Autodesk Fusion 360 part; units mm, degrees
(part 16 of 21)
extrude "Estrusione10" add sketch "Schizzo9" along normal blind 1 text T0 in component "Spur Gear (60 teeth) (1)"
component "Spur Gear (60 teeth) (1)" placed x (1, 0, 0) y (0, 1, 0) z (0, 0, 1) at (0, 0, 0)

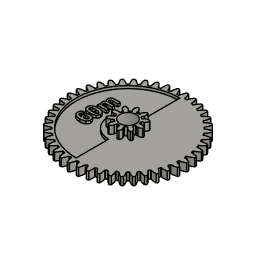
design "6 intermedio ore"
description: Spur Gear; Module: 1.000000; Num Teeth: 44; Pressure Angle: 20.000000; Backlash: 0.00 mm
description: Spur Gear; Module: 1.000000; Num Teeth: 10; Pressure Angle: 20.000000; Backlash: 0.00 mm
Autodesk Fusion 360 part; units mm, degrees
sketch "Schizzo1" plane through (0, 0, 0) normal (0, 0, 1) x (1, 0, 0) in component "Spur Gear (44 teeth)"
  circle A0 centre (0, 0) radius 20.7492
  circle A1 centre (0, 0) radius 3.1
extrude "Estrusione1" add sketch "Schizzo1" along normal blind 3 makes body 1 in component "Spur Gear (44 teeth)"
sketch "Schizzo2" plane through (0, 0, 0) normal (0, 0, 1) x (1, 0, 0) in component "Spur Gear (44 teeth)"
  spline S0 degree 5 poles (20.6468, -1.0457) (20.6535, -1.0457) (20.667, -1.0458) (20.6873, -1.0456) (20.7143, -1.0451) (20.7481, -1.044) (20.7819, -1.0422) (20.8157, -1.04) (20.8495, -1.0372) (20.8833, -1.034) (20.9172, -1.0304) (20.951, -1.0264) (20.9848, -1.022) (21.0187, -1.0174) (21.0525, -1.0125) (21.0863, -1.0073) (21.1202, -1.0019) (21.154, -0.9961) (21.1878, -0.9902) (21.2216, -0.9839) (21.2554, -0.9774) (21.2892, -0.9707) (21.323, -0.9637) (21.3568, -0.9565) (21.3906, -0.9491) (21.4244, -0.9415) (21.4581, -0.9337) (21.4919, -0.9256) (21.5256, -0.9174) (21.5594, -0.9089) (21.5931, -0.9002) (21.6268, -0.8914) (21.6605, -0.8823) (21.6942, -0.8731) (21.7279, -0.8636) (21.7616, -0.854) (21.7952, -0.8442) (21.8289, -0.8343) (21.8625, -0.8241) (21.8961, -0.8138) (21.9298, -0.8033) (21.9634, -0.7926) (21.9969, -0.7817) (22.0305, -0.7707) (22.0641, -0.7595) (22.0976, -0.7481) (22.1311, -0.7366) (22.1646, -0.7249) (22.1981, -0.7131) (22.2316, -0.7011) (22.2651, -0.6889) (22.2985, -0.6766) (22.332, -0.6642) (22.3654, -0.6515) (22.3988, -0.6387) (22.4322, -0.6258) (22.4655, -0.6127) (22.4989, -0.5995) (22.5322, -0.5861) (22.5655, -0.5726) (22.5988, -0.5589) (22.6321, -0.5451) (22.6653, -0.5311) (22.6986, -0.517) (22.7318, -0.5027) (22.765, -0.4883) (22.7982, -0.4738) (22.8313, -0.4591) (22.8645, -0.4443) (22.8976, -0.4294) (22.9307, -0.4143) (22.9571, -0.4021) (22.977, -0.3929) (22.9902, -0.3867) (22.9968, -0.3836) knots 0 0 0 0 0 0 0.01428571 0.02857143 0.04285714 0.05714286 0.07142857 0.08571429 0.1 0.11428571 0.12857143 0.14285714 0.15714286 0.17142857 0.18571429 0.2 0.21428571 0.22857143 0.24285714 0.25714286 0.27142857 0.28571429 0.3 0.31428571 0.32857143 0.34285714 0.35714286 0.37142857 0.38571429 0.4 0.41428571 0.42857143 0.44285714 0.45714286 0.47142857 0.48571429 0.5 0.51428571 0.52857143 0.54285714 0.55714286 0.57142857 0.58571429 0.6 0.61428571 0.62857143 0.64285714 0.65714286 0.67142857 0.68571429 0.7 0.71428571 0.72857143 0.74285714 0.75714286 0.77142857 0.78571429 0.8 0.81428571 0.82857143 0.84285714 0.85714286 0.87142857 0.88571429 0.9 0.91428571 0.92857143 0.94285714 0.95714286 0.97142857 0.98571429 1 1 1 1 1 1
  spline S1 degree 5 poles (20.6468, 1.0457) (20.6535, 1.0457) (20.667, 1.0458) (20.6873, 1.0456) (20.7143, 1.0451) (20.7481, 1.044) (20.7819, 1.0422) (20.8157, 1.04) (20.8495, 1.0372) (20.8833, 1.034) (20.9172, 1.0304) (20.951, 1.0264) (20.9848, 1.022) (21.0187, 1.0174) (21.0525, 1.0125) (21.0863, 1.0073) (21.1202, 1.0019) (21.154, 0.9961) (21.1878, 0.9902) (21.2216, 0.9839) (21.2554, 0.9774) (21.2892, 0.9707) (21.323, 0.9637) (21.3568, 0.9565) (21.3906, 0.9491) (21.4244, 0.9415) (21.4581, 0.9337) (21.4919, 0.9256) (21.5256, 0.9174) (21.5594, 0.9089) (21.5931, 0.9002) (21.6268, 0.8914) (21.6605, 0.8823) (21.6942, 0.8731) (21.7279, 0.8636) (21.7616, 0.854) (21.7952, 0.8442) (21.8289, 0.8343) (21.8625, 0.8241) (21.8961, 0.8138) (21.9298, 0.8033) (21.9634, 0.7926) (21.9969, 0.7817) (22.0305, 0.7707) (22.0641, 0.7595) (22.0976, 0.7481) (22.1311, 0.7366) (22.1646, 0.7249) (22.1981, 0.7131) (22.2316, 0.7011) (22.2651, 0.6889) (22.2985, 0.6766) (22.332, 0.6642) (22.3654, 0.6515) (22.3988, 0.6387) (22.4322, 0.6258) (22.4655, 0.6127) (22.4989, 0.5995) (22.5322, 0.5861) (22.5655, 0.5726) (22.5988, 0.5589) (22.6321, 0.5451) (22.6653, 0.5311) (22.6986, 0.517) (22.7318, 0.5027) (22.765, 0.4883) (22.7982, 0.4738) (22.8313, 0.4591) (22.8645, 0.4443) (22.8976, 0.4294) (22.9307, 0.4143) (22.9571, 0.4021) (22.977, 0.3929) (22.9902, 0.3867) (22.9968, 0.3836) knots 0 0 0 0 0 0 0.01428571 0.02857143 0.04285714 0.05714286 0.07142857 0.08571429 0.1 0.11428571 0.12857143 0.14285714 0.15714286 0.17142857 0.18571429 0.2 0.21428571 0.22857143 0.24285714 0.25714286 0.27142857 0.28571429 0.3 0.31428571 0.32857143 0.34285714 0.35714286 0.37142857 0.38571429 0.4 0.41428571 0.42857143 0.44285714 0.45714286 0.47142857 0.48571429 0.5 0.51428571 0.52857143 0.54285714 0.55714286 0.57142857 0.58571429 0.6 0.61428571 0.62857143 0.64285714 0.65714286 0.67142857 0.68571429 0.7 0.71428571 0.72857143 0.74285714 0.75714286 0.77142857 0.78571429 0.8 0.81428571 0.82857143 0.84285714 0.85714286 0.87142857 0.88571429 0.9 0.91428571 0.92857143 0.94285714 0.95714286 0.97142857 0.98571429 1 1 1 1 1 1
  arc A0 (22.9968, -0.3836) -> (22.9968, 0.3836) centre (0, 0) ccw
  line L0 (20.6468, 1.0457) -> (20.6468, -1.0457)
  point P0 (20.8135, -1.04)
  point P1 (20.9807, -1.0225)
  point P2 (21.1483, -0.9971)
  point P3 (21.3162, -0.9651)
  point P4 (21.4842, -0.9274)
  point P5 (21.6524, -0.8845)
  point P6 (21.8206, -0.8367)
  point P7 (21.9888, -0.7843)
  point P8 (22.1571, -0.7276)
  point P9 (22.3253, -0.6666)
  point P10 (22.4934, -0.6017)
  point P11 (22.6613, -0.5328)
  point P12 (22.8292, -0.4601)
  point P13 (20.8135, 1.04)
  point P14 (20.9807, 1.0225)
  point P15 (21.1483, 0.9971)
  point P16 (21.3162, 0.9651)
  point P17 (21.4842, 0.9274)
  point P18 (21.6524, 0.8845)
  point P19 (21.8206, 0.8367)
  point P20 (21.9888, 0.7843)
  point P21 (22.1571, 0.7276)
  point P22 (22.3253, 0.6666)
  point P23 (22.4934, 0.6017)
  point P24 (22.6613, 0.5328)
  point P25 (22.8292, 0.4601)
extrude "Estrusione2" add sketch "Schizzo2" along normal blind 3 bodies 1 in component "Spur Gear (44 teeth)"
fillet "Raccordo1" radius 0.1 2 edges at (20.7229, 1.0448, 1.5) (20.7229, -1.0448, 1.5) on bodies 1 in component "Spur Gear (44 teeth)"
pattern_circular "Serie C1" count 44 over 360 about axis through (0, 0, 0) along (0, 0, 1) of "Estrusione2", "Raccordo1" in component "Spur Gear (44 teeth)"
sketch "Schizzo3" plane through (0, 0, 0) normal (0, 0, 1) x (1, 0, 0) in component "Spur Gear (44 teeth)"
  circle A0 centre (0, 0) radius 22 construction
sketch "Schizzo1 (2)" plane through (0, 0, 0) normal (0, 0, 1) x (1, 0, 0) in component "Spur Gear (10 teeth)"
  circle A0 centre (0, 0) radius 3.7492
  circle A1 centre (0, 0) radius 3.1
extrude "Estrusione1'" add sketch "Schizzo1 (2)" along normal blind 6 separate body makes body 2 in component "Spur Gear (10 teeth)"
sketch "Schizzo2 (2)" plane through (0, 0, 0) normal (0, 0, 1) x (1, 0, 0) in component "Spur Gear (10 teeth)"
  spline S0 degree 5 poles (4.6291, -0.8041) (4.6329, -0.8047) (4.6405, -0.8059) (4.6519, -0.8073) (4.6672, -0.8084) (4.6864, -0.8088) (4.7057, -0.8085) (4.7251, -0.8077) (4.7445, -0.8066) (4.7639, -0.8054) (4.7834, -0.804) (4.8029, -0.8024) (4.8224, -0.8004) (4.842, -0.7981) (4.8616, -0.7954) (4.8812, -0.7924) (4.9009, -0.7891) (4.9205, -0.7856) (4.9402, -0.7818) (4.9599, -0.7778) (4.9796, -0.7737) (4.9993, -0.7693) (5.019, -0.7646) (5.0388, -0.7598) (5.0585, -0.7547) (5.0783, -0.7493) (5.098, -0.7438) (5.1178, -0.738) (5.1375, -0.7321) (5.1573, -0.7259) (5.177, -0.7196) (5.1968, -0.7131) (5.2165, -0.7063) (5.2363, -0.6994) (5.256, -0.6923) (5.2757, -0.685) (5.2955, -0.6775) (5.3152, -0.6698) (5.3349, -0.6619) (5.3546, -0.6538) (5.3743, -0.6456) (5.394, -0.6372) (5.4136, -0.6286) (5.4333, -0.6198) (5.4529, -0.6109) (5.4725, -0.6018) (5.4921, -0.5925) (5.5117, -0.583) (5.5312, -0.5734) (5.5508, -0.5636) (5.5703, -0.5536) (5.5898, -0.5435) (5.6093, -0.5332) (5.6287, -0.5228) (5.6482, -0.5121) (5.6676, -0.5013) (5.6869, -0.4904) (5.7063, -0.4793) (5.7256, -0.468) (5.7449, -0.4566) (5.7642, -0.445) (5.7834, -0.4332) (5.8026, -0.4213) (5.8218, -0.4093) (5.8409, -0.397) (5.86, -0.3847) (5.8791, -0.3721) (5.8982, -0.3595) (5.9172, -0.3466) (5.9361, -0.3336) (5.9551, -0.3205) (5.9702, -0.3099) (5.9815, -0.3018) (5.989, -0.2964) (5.9928, -0.2937) knots 0 0 0 0 0 0 0.01428571 0.02857143 0.04285714 0.05714286 0.07142857 0.08571429 0.1 0.11428571 0.12857143 0.14285714 0.15714286 0.17142857 0.18571429 0.2 0.21428571 0.22857143 0.24285714 0.25714286 0.27142857 0.28571429 0.3 0.31428571 0.32857143 0.34285714 0.35714286 0.37142857 0.38571429 0.4 0.41428571 0.42857143 0.44285714 0.45714286 0.47142857 0.48571429 0.5 0.51428571 0.52857143 0.54285714 0.55714286 0.57142857 0.58571429 0.6 0.61428571 0.62857143 0.64285714 0.65714286 0.67142857 0.68571429 0.7 0.71428571 0.72857143 0.74285714 0.75714286 0.77142857 0.78571429 0.8 0.81428571 0.82857143 0.84285714 0.85714286 0.87142857 0.88571429 0.9 0.91428571 0.92857143 0.94285714 0.95714286 0.97142857 0.98571429 1 1 1 1 1 1
  spline S1 degree 5 poles (4.6291, 0.8041) (4.6329, 0.8047) (4.6405, 0.8059) (4.6519, 0.8073) (4.6672, 0.8084) (4.6864, 0.8088) (4.7057, 0.8085) (4.7251, 0.8077) (4.7445, 0.8066) (4.7639, 0.8054) (4.7834, 0.804) (4.8029, 0.8024) (4.8224, 0.8004) (4.842, 0.7981) (4.8616, 0.7954) (4.8812, 0.7924) (4.9009, 0.7891) (4.9205, 0.7856) (4.9402, 0.7818) (4.9599, 0.7778) (4.9796, 0.7737) (4.9993, 0.7693) (5.019, 0.7646) (5.0388, 0.7598) (5.0585, 0.7547) (5.0783, 0.7493) (5.098, 0.7438) (5.1178, 0.738) (5.1375, 0.7321) (5.1573, 0.7259) (5.177, 0.7196) (5.1968, 0.7131) (5.2165, 0.7063) (5.2363, 0.6994) (5.256, 0.6923) (5.2757, 0.685) (5.2955, 0.6775) (5.3152, 0.6698) (5.3349, 0.6619) (5.3546, 0.6538) (5.3743, 0.6456) (5.394, 0.6372) (5.4136, 0.6286) (5.4333, 0.6198) (5.4529, 0.6109) (5.4725, 0.6018) (5.4921, 0.5925) (5.5117, 0.583) (5.5312, 0.5734) (5.5508, 0.5636) (5.5703, 0.5536) (5.5898, 0.5435) (5.6093, 0.5332) (5.6287, 0.5228) (5.6482, 0.5121) (5.6676, 0.5013) (5.6869, 0.4904) (5.7063, 0.4793) (5.7256, 0.468) (5.7449, 0.4566) (5.7642, 0.445) (5.7834, 0.4332) (5.8026, 0.4213) (5.8218, 0.4093) (5.8409, 0.397) (5.86, 0.3847) (5.8791, 0.3721) (5.8982, 0.3595) (5.9172, 0.3466) (5.9361, 0.3336) (5.9551, 0.3205) (5.9702, 0.3099) (5.9815, 0.3018) (5.989, 0.2964) (5.9928, 0.2937) knots 0 0 0 0 0 0 0.01428571 0.02857143 0.04285714 0.05714286 0.07142857 0.08571429 0.1 0.11428571 0.12857143 0.14285714 0.15714286 0.17142857 0.18571429 0.2 0.21428571 0.22857143 0.24285714 0.25714286 0.27142857 0.28571429 0.3 0.31428571 0.32857143 0.34285714 0.35714286 0.37142857 0.38571429 0.4 0.41428571 0.42857143 0.44285714 0.45714286 0.47142857 0.48571429 0.5 0.51428571 0.52857143 0.54285714 0.55714286 0.57142857 0.58571429 0.6 0.61428571 0.62857143 0.64285714 0.65714286 0.67142857 0.68571429 0.7 0.71428571 0.72857143 0.74285714 0.75714286 0.77142857 0.78571429 0.8 0.81428571 0.82857143 0.84285714 0.85714286 0.87142857 0.88571429 0.9 0.91428571 0.92857143 0.94285714 0.95714286 0.97142857 0.98571429 1 1 1 1 1 1
  arc A0 (5.9928, -0.2937) -> (5.9928, 0.2937) centre (0, 0) ccw
  line L0 (3.684, -0.6416) -> (4.6291, -0.8041)
  line L1 (3.684, 0.6416) -> (4.6291, 0.8041)
  line L2 (3.684, -0.6416) -> (3.684, 0.6416)
  point P0 (4.7229, -0.8077)
  point P1 (4.8183, -0.8008)
  point P2 (4.9148, -0.7866)
  point P3 (5.0121, -0.7662)
  point P4 (5.11, -0.7403)
  point P5 (5.2082, -0.7091)
  point P6 (5.3067, -0.673)
  point P7 (5.4054, -0.6322)
  point P8 (5.504, -0.5867)
  point P9 (5.6025, -0.5368)
  point P10 (5.7007, -0.4824)
  point P11 (5.7986, -0.4238)
  point P12 (5.896, -0.3609)
  point P13 (4.7229, 0.8077)
  point P14 (4.8183, 0.8008)
  point P15 (4.9148, 0.7866)
  point P16 (5.0121, 0.7662)
  point P17 (5.11, 0.7403)
  point P18 (5.2082, 0.7091)
  point P19 (5.3067, 0.673)
  point P20 (5.4054, 0.6322)
  point P21 (5.504, 0.5867)
  point P22 (5.6025, 0.5368)
  point P23 (5.7007, 0.4824)
  point P24 (5.7986, 0.4238)
  point P25 (5.896, 0.3609)
extrude "Estrusione2'" add sketch "Schizzo2 (2)" along normal blind 6 bodies 2 in component "Spur Gear (10 teeth)"
fillet "Raccordo1'" radius 0.1 2 edges at (3.6936, -0.6433, 3) (3.6936, 0.6433, 3) on bodies 2 in component "Spur Gear (10 teeth)"
pattern_circular "Serie C1'" count 10 over 360 about axis through (0, 0, 0) along (0, 0, 1) of "Estrusione2'", "Raccordo1'" in component "Spur Gear (10 teeth)"
sketch "Schizzo3 (2)" plane through (0, 0, 0) normal (0, 0, 1) x (1, 0, 0) in component "Spur Gear (10 teeth)"
  circle A0 centre (0, 0) radius 5 construction
combine "Combina1" operation add target body 1 tool bodies 2 in component "Spur Gear (44 teeth)"
sketch "Schizzo1 (3)" plane through (0, 0, 3) normal (0, 0, 1) x (-1, 0, 0)
  arc A0 (-3.7907, 0.66) -> (-3.6757, 0.7388) centre (-3.7737, 0.7585) ccw
  arc A1 (-3.408, 1.5628) -> (-3.6757, 0.7388) centre (0, 0) ccw
  arc A2 (-3.408, 1.5628) -> (-3.4546, 1.6942) centre (-3.4988, 1.6045) ccw
  line L0 (-3.4546, 1.6942) -> (-4.2177, 2.0704)
  spline S0 degree 3 poles (-4.2177, 2.0704) (-4.2458, 2.0843) (-4.2713, 2.1025) (-4.3719, 2.1848) (-4.5424, 2.3303) (-4.8488, 2.838) (-4.9461, 3.0593) (-5.0209, 3.2848) knots 0 0 0 0 0.009402 0.009402 0.024238 0.024238 0.034093 0.034093 0.034093 0.034093
  arc A3 (-4.6756, 3.7601) -> (-5.0209, 3.2848) centre (0, 0) ccw
  spline S1 degree 3 poles (-4.6756, 3.7601) (-4.4172, 3.7585) (-4.1552, 3.7302) (-3.7444, 3.6242) (-3.6325, 3.5789) (-3.4729, 3.5079) (-3.34, 3.4408) (-3.2724, 3.3715) knots 0 0 0 0 0.077518 0.077518 0.128006 0.128006 0.19629 0.19629 0.19629 0.19629
  line L1 (-3.2724, 3.3715) -> (-2.6788, 2.762)
  arc A4 (-2.6788, 2.762) -> (-2.5394, 2.7582) centre (-2.6072, 2.8318) ccw
  arc A5 (-1.8385, 3.2675) -> (-2.5394, 2.7582) centre (0, 0) ccw
  arc A6 (-1.8385, 3.2675) -> (-1.799, 3.4012) centre (-1.8875, 3.3546) ccw
  line L2 (-1.799, 3.4012) -> (-2.1952, 4.1541)
  spline S2 degree 3 poles (-2.1952, 4.1541) (-2.2098, 4.1818) (-2.2197, 4.2116) (-2.2528, 4.3373) (-2.3052, 4.5552) (-2.2547, 5.1461) (-2.2033, 5.3822) (-2.1312, 5.6087) knots 0 0 0 0 0.009402 0.009402 0.024238 0.024238 0.034093 0.034093 0.034093 0.034093
  arc A7 (-1.5725, 5.7903) -> (-2.1312, 5.6087) centre (0, 0) ccw
  spline S3 degree 3 poles (-1.5725, 5.7903) (-1.3644, 5.6371) (-1.1691, 5.4601) (-0.899, 5.133) (-0.8351, 5.0306) (-0.7478, 4.8792) (-0.6796, 4.7468) (-0.6658, 4.6511) knots 0 0 0 0 0.077518 0.077518 0.128006 0.128006 0.19629 0.19629 0.19629 0.19629
  line L3 (-0.6658, 4.6511) -> (-0.5437, 3.8091)
  arc A8 (-0.5437, 3.8091) -> (-0.4332, 3.7241) centre (-0.4448, 3.8234) ccw
  arc A9 (0.4332, 3.7241) -> (-0.4332, 3.7241) centre (0, 0) ccw
  arc A10 (0.4332, 3.7241) -> (0.5437, 3.8091) centre (0.4448, 3.8234) ccw
  line L4 (0.5437, 3.8091) -> (0.6658, 4.6511)
  spline S4 degree 3 poles (0.6658, 4.6511) (0.6703, 4.6821) (0.6797, 4.7119) (0.7268, 4.8331) (0.8125, 5.0402) (1.2007, 5.4885) (1.3811, 5.6494) (1.5725, 5.7903) knots 0 0 0 0 0.009402 0.009402 0.024238 0.024238 0.034093 0.034093 0.034093 0.034093
  arc A11 (2.1312, 5.6087) -> (1.5725, 5.7903) centre (0, 0) ccw
  spline S5 degree 3 poles (2.1312, 5.6087) (2.2096, 5.3625) (2.2636, 5.1045) (2.2897, 4.6811) (2.2813, 4.5607) (2.263, 4.3869) (2.2403, 4.2397) (2.1952, 4.1541) knots 0 0 0 0 0.077518 0.077518 0.128006 0.128006 0.19629 0.19629 0.19629 0.19629
  line L5 (2.1952, 4.1541) -> (1.799, 3.4012)
  arc A12 (1.799, 3.4012) -> (1.8385, 3.2675) centre (1.8875, 3.3546) ccw
  arc A13 (2.5394, 2.7582) -> (1.8385, 3.2675) centre (0, 0) ccw
  arc A14 (2.5394, 2.7582) -> (2.6788, 2.762) centre (2.6072, 2.8318) ccw
  line L6 (2.6788, 2.762) -> (3.2724, 3.3715)
  spline S6 degree 3 poles (3.2724, 3.3715) (3.2943, 3.3939) (3.3195, 3.4125) (3.4288, 3.4828) (3.6199, 3.6) (4.1975, 3.7345) (4.438, 3.7587) (4.6756, 3.7601) knots 0 0 0 0 0.009402 0.009402 0.024238 0.024238 0.034093 0.034093 0.034093 0.034093
  arc A15 (5.0209, 3.2848) -> (4.6756, 3.7601) centre (0, 0) ccw
  spline S7 degree 3 poles (5.0209, 3.2848) (4.9396, 3.0396) (4.8316, 2.7991) (4.6039, 2.4412) (4.5263, 2.3488) (4.4094, 2.2189) (4.3045, 2.1132) (4.2177, 2.0704) knots 0 0 0 0 0.077518 0.077518 0.128006 0.128006 0.19629 0.19629 0.19629 0.19629
  line L7 (4.2177, 2.0704) -> (3.4546, 1.6942)
  arc A16 (3.4546, 1.6942) -> (3.408, 1.5628) centre (3.4988, 1.6045) ccw
  arc A17 (3.6757, 0.7388) -> (3.408, 1.5628) centre (0, 0) ccw
  arc A18 (3.6757, 0.7388) -> (3.7907, 0.66) centre (3.7737, 0.7585) ccw
  line L8 (3.7907, 0.66) -> (4.6291, 0.8041)
  spline S8 degree 3 poles (4.6291, 0.8041) (4.66, 0.8094) (4.6914, 0.8096) (4.8211, 0.8023) (5.0446, 0.7847) (5.5909, 0.5541) (5.7997, 0.4323) (5.9928, 0.2937) knots 0 0 0 0 0.009402 0.009402 0.024238 0.024238 0.034093 0.034093 0.034093 0.034093
  arc A19 (5.9928, -0.2937) -> (5.9928, 0.2937) centre (0, 0) ccw
  spline S9 degree 3 poles (5.9928, -0.2937) (5.7828, -0.4443) (5.5541, -0.5754) (5.1596, -0.7311) (5.0424, -0.7603) (4.8715, -0.7966) (4.7245, -0.8205) (4.6291, -0.8041) knots 0 0 0 0 0.077518 0.077518 0.128006 0.128006 0.19629 0.19629 0.19629 0.19629
  line L9 (4.6291, -0.8041) -> (3.7907, -0.66)
  arc A20 (3.7907, -0.66) -> (3.6757, -0.7388) centre (3.7737, -0.7585) ccw
  arc A21 (3.408, -1.5628) -> (3.6757, -0.7388) centre (0, 0) ccw
  arc A22 (3.408, -1.5628) -> (3.4546, -1.6942) centre (3.4988, -1.6045) ccw
  line L10 (3.4546, -1.6942) -> (4.2177, -2.0704)
  spline S10 degree 3 poles (4.2177, -2.0704) (4.2458, -2.0843) (4.2713, -2.1025) (4.3719, -2.1848) (4.5424, -2.3303) (4.8488, -2.838) (4.9461, -3.0593) (5.0209, -3.2848) knots 0 0 0 0 0.009402 0.009402 0.024238 0.024238 0.034093 0.034093 0.034093 0.034093
  arc A23 (4.6756, -3.7601) -> (5.0209, -3.2848) centre (0, 0) ccw
  spline S11 degree 3 poles (4.6756, -3.7601) (4.4172, -3.7585) (4.1552, -3.7302) (3.7444, -3.6242) (3.6325, -3.5789) (3.4729, -3.5079) (3.34, -3.4408) (3.2724, -3.3715) knots 0 0 0 0 0.077518 0.077518 0.128006 0.128006 0.19629 0.19629 0.19629 0.19629
  line L11 (3.2724, -3.3715) -> (2.6788, -2.762)
  arc A24 (2.6788, -2.762) -> (2.5394, -2.7582) centre (2.6072, -2.8318) ccw
  arc A25 (1.8385, -3.2675) -> (2.5394, -2.7582) centre (0, 0) ccw
  arc A26 (1.8385, -3.2675) -> (1.799, -3.4012) centre (1.8875, -3.3546) ccw
  line L12 (1.799, -3.4012) -> (2.1952, -4.1541)
  spline S12 degree 3 poles (2.1952, -4.1541) (2.2098, -4.1818) (2.2197, -4.2116) (2.2528, -4.3373) (2.3052, -4.5552) (2.2547, -5.1461) (2.2033, -5.3822) (2.1312, -5.6087) knots 0 0 0 0 0.009402 0.009402 0.024238 0.024238 0.034093 0.034093 0.034093 0.034093
  arc A27 (1.5725, -5.7903) -> (2.1312, -5.6087) centre (0, 0) ccw
  spline S13 degree 3 poles (1.5725, -5.7903) (1.3644, -5.6371) (1.1691, -5.4601) (0.899, -5.133) (0.8351, -5.0306) (0.7478, -4.8792) (0.6796, -4.7468) (0.6658, -4.6511) knots 0 0 0 0 0.077518 0.077518 0.128006 0.128006 0.19629 0.19629 0.19629 0.19629
  line L13 (0.6658, -4.6511) -> (0.5437, -3.8091)
  arc A28 (0.5437, -3.8091) -> (0.4332, -3.7241) centre (0.4448, -3.8234) ccw
  arc A29 (-0.4332, -3.7241) -> (0.4332, -3.7241) centre (0, 0) ccw
  arc A30 (-0.4332, -3.7241) -> (-0.5437, -3.8091) centre (-0.4448, -3.8234) ccw
  line L14 (-0.5437, -3.8091) -> (-0.6658, -4.6511)
  spline S14 degree 3 poles (-0.6658, -4.6511) (-0.6703, -4.6821) (-0.6797, -4.7119) (-0.7268, -4.8331) (-0.8125, -5.0402) (-1.2007, -5.4885) (-1.3811, -5.6494) (-1.5725, -5.7903) knots 0 0 0 0 0.009402 0.009402 0.024238 0.024238 0.034093 0.034093 0.034093 0.034093
  arc A31 (-2.1312, -5.6087) -> (-1.5725, -5.7903) centre (0, 0) ccw
  spline S15 degree 3 poles (-2.1312, -5.6087) (-2.2096, -5.3625) (-2.2636, -5.1045) (-2.2897, -4.6811) (-2.2813, -4.5607) (-2.263, -4.3869) (-2.2403, -4.2397) (-2.1952, -4.1541) knots 0 0 0 0 0.077518 0.077518 0.128006 0.128006 0.19629 0.19629 0.19629 0.19629
  line L15 (-2.1952, -4.1541) -> (-1.799, -3.4012)
  arc A32 (-1.799, -3.4012) -> (-1.8385, -3.2675) centre (-1.8875, -3.3546) ccw
  arc A33 (-2.5394, -2.7582) -> (-1.8385, -3.2675) centre (0, 0) ccw
  arc A34 (-2.5394, -2.7582) -> (-2.6788, -2.762) centre (-2.6072, -2.8318) ccw
  line L16 (-2.6788, -2.762) -> (-3.2724, -3.3715)
  spline S16 degree 3 poles (-3.2724, -3.3715) (-3.2943, -3.3939) (-3.3195, -3.4125) (-3.4288, -3.4828) (-3.6199, -3.6) (-4.1975, -3.7345) (-4.438, -3.7587) (-4.6756, -3.7601) knots 0 0 0 0 0.009402 0.009402 0.024238 0.024238 0.034093 0.034093 0.034093 0.034093
  arc A35 (-5.0209, -3.2848) -> (-4.6756, -3.7601) centre (0, 0) ccw
  spline S17 degree 3 poles (-5.0209, -3.2848) (-4.9396, -3.0396) (-4.8316, -2.7991) (-4.6039, -2.4412) (-4.5263, -2.3488) (-4.4094, -2.2189) (-4.3045, -2.1132) (-4.2177, -2.0704) knots 0 0 0 0 0.077518 0.077518 0.128006 0.128006 0.19629 0.19629 0.19629 0.19629
  line L17 (-4.2177, -2.0704) -> (-3.4546, -1.6942)
  arc A36 (-3.4546, -1.6942) -> (-3.408, -1.5628) centre (-3.4988, -1.6045) ccw
  arc A37 (-3.6757, -0.7388) -> (-3.408, -1.5628) centre (0, 0) ccw
  arc A38 (-3.6757, -0.7388) -> (-3.7907, -0.66) centre (-3.7737, -0.7585) ccw
  line L18 (-3.7907, -0.66) -> (-4.6291, -0.8041)
  spline S18 degree 3 poles (-4.6291, -0.8041) (-4.66, -0.8094) (-4.6914, -0.8096) (-4.8211, -0.8023) (-5.0446, -0.7847) (-5.5909, -0.5541) (-5.7997, -0.4323) (-5.9928, -0.2937) knots 0 0 0 0 0.009402 0.009402 0.024238 0.024238 0.034093 0.034093 0.034093 0.034093
  arc A39 (-5.9928, 0.2937) -> (-5.9928, -0.2937) centre (0, 0) ccw
  spline S19 degree 3 poles (-5.9928, 0.2937) (-5.7828, 0.4443) (-5.5541, 0.5754) (-5.1596, 0.7311) (-5.0424, 0.7603) (-4.8715, 0.7966) (-4.7245, 0.8205) (-4.6291, 0.8041) knots 0 0 0 0 0.077518 0.077518 0.128006 0.128006 0.19629 0.19629 0.19629 0.19629
  line L19 (-4.6291, 0.8041) -> (-3.7907, 0.66)
  arc A40 (-20.6687, 1.8256) -> (-20.7182, 1.1345) centre (0, 0) ccw
  spline S20 degree 3 poles (-20.8108, 1.0402) (-20.7979, 1.0411) (-20.7852, 1.0446) (-20.7619, 1.0562) (-20.7514, 1.0642) (-20.7355, 1.0824) (-20.7296, 1.0919) (-20.7212, 1.1125) (-20.7188, 1.1234) (-20.7182, 1.1345) knots 0 0 0 0 0.003906 0.003906 0.007813 0.007813 0.011148 0.011148 0.014483 0.014483 0.014483 0.014483
  spline S21 degree 5 poles (-20.8108, 1.0402) (-20.8118, 1.0401) (-20.8195, 1.0396) (-20.834, 1.0385) (-20.8553, 1.0367) (-20.8833, 1.034) (-20.9172, 1.0304) (-20.951, 1.0264) (-20.9848, 1.022) (-21.0187, 1.0174) (-21.0525, 1.0125) (-21.0863, 1.0073) (-21.1202, 1.0019) (-21.154, 0.9961) (-21.1878, 0.9902) (-21.2216, 0.9839) (-21.2554, 0.9774) (-21.2892, 0.9707) (-21.323, 0.9637) (-21.3568, 0.9565) (-21.3906, 0.9491) (-21.4244, 0.9415) (-21.4581, 0.9337) (-21.4919, 0.9256) (-21.5256, 0.9174) (-21.5594, 0.9089) (-21.5931, 0.9002) (-21.6268, 0.8914) (-21.6605, 0.8823) (-21.6942, 0.8731) (-21.7279, 0.8636) (-21.7616, 0.854) (-21.7952, 0.8442) (-21.8289, 0.8343) (-21.8625, 0.8241) (-21.8961, 0.8138) (-21.9298, 0.8033) (-21.9634, 0.7926) (-21.9969, 0.7817) (-22.0305, 0.7707) (-22.0641, 0.7595) (-22.0976, 0.7481) (-22.1311, 0.7366) (-22.1646, 0.7249) (-22.1981, 0.7131) (-22.2316, 0.7011) (-22.2651, 0.6889) (-22.2985, 0.6766) (-22.332, 0.6642) (-22.3654, 0.6515) (-22.3988, 0.6387) (-22.4322, 0.6258) (-22.4655, 0.6127) (-22.4989, 0.5995) (-22.5322, 0.5861) (-22.5655, 0.5726) (-22.5988, 0.5589) (-22.6321, 0.5451) (-22.6653, 0.5311) (-22.6986, 0.517) (-22.7318, 0.5027) (-22.765, 0.4883) (-22.7982, 0.4738) (-22.8313, 0.4591) (-22.8645, 0.4443) (-22.8976, 0.4294) (-22.9307, 0.4143) (-22.9571, 0.4021) (-22.977, 0.3929) (-22.9902, 0.3867) (-22.9968, 0.3836) knots 0.06937658 0.06937658 0.06937658 0.06937658 0.06937658 0.06937658 0.07142857 0.08571429 0.1 0.11428571 0.12857143 0.14285714 0.15714286 0.17142857 0.18571429 0.2 0.21428571 0.22857143 0.24285714 0.25714286 0.27142857 0.28571429 0.3 0.31428571 0.32857143 0.34285714 0.35714286 0.37142857 0.38571429 0.4 0.41428571 0.42857143 0.44285714 0.45714286 0.47142857 0.48571429 0.5 0.51428571 0.52857143 0.54285714 0.55714286 0.57142857 0.58571429 0.6 0.61428571 0.62857143 0.64285714 0.65714286 0.67142857 0.68571429 0.7 0.71428571 0.72857143 0.74285714 0.75714286 0.77142857 0.78571429 0.8 0.81428571 0.82857143 0.84285714 0.85714286 0.87142857 0.88571429 0.9 0.91428571 0.92857143 0.94285714 0.95714286 0.97142857 0.98571429 1 1 1 1 1 1
  arc A41 (-22.9968, 0.3836) -> (-22.9968, -0.3836) centre (0, 0) ccw
  spline S22 degree 5 poles (-22.9968, -0.3836) (-22.9902, -0.3867) (-22.977, -0.3929) (-22.9571, -0.4021) (-22.9307, -0.4143) (-22.8976, -0.4294) (-22.8645, -0.4443) (-22.8313, -0.4591) (-22.7982, -0.4738) (-22.765, -0.4883) (-22.7318, -0.5027) (-22.6986, -0.517) (-22.6653, -0.5311) (-22.6321, -0.5451) (-22.5988, -0.5589) (-22.5655, -0.5726) (-22.5322, -0.5861) (-22.4989, -0.5995) (-22.4655, -0.6127) (-22.4322, -0.6258) (-22.3988, -0.6387) (-22.3654, -0.6515) (-22.332, -0.6642) (-22.2985, -0.6766) (-22.2651, -0.6889) (-22.2316, -0.7011) (-22.1981, -0.7131) (-22.1646, -0.7249) (-22.1311, -0.7366) (-22.0976, -0.7481) (-22.0641, -0.7595) (-22.0305, -0.7707) (-21.9969, -0.7817) (-21.9634, -0.7926) (-21.9298, -0.8033) (-21.8961, -0.8138) (-21.8625, -0.8241) (-21.8289, -0.8343) (-21.7952, -0.8442) (-21.7616, -0.854) (-21.7279, -0.8636) (-21.6942, -0.8731) (-21.6605, -0.8823) (-21.6268, -0.8914) (-21.5931, -0.9002) (-21.5594, -0.9089) (-21.5256, -0.9174) (-21.4919, -0.9256) (-21.4581, -0.9337) (-21.4244, -0.9415) (-21.3906, -0.9491) (-21.3568, -0.9565) (-21.323, -0.9637) (-21.2892, -0.9707) (-21.2554, -0.9774) (-21.2216, -0.9839) (-21.1878, -0.9902) (-21.154, -0.9961) (-21.1202, -1.0019) (-21.0863, -1.0073) (-21.0525, -1.0125) (-21.0187, -1.0174) (-20.9848, -1.022) (-20.951, -1.0264) (-20.9172, -1.0304) (-20.8833, -1.034) (-20.8553, -1.0367) (-20.834, -1.0385) (-20.8195, -1.0396) (-20.8118, -1.0401) (-20.8108, -1.0402) knots -1 -1 -1 -1 -1 -1 -0.98571429 -0.97142857 -0.95714286 -0.94285714 -0.92857143 -0.91428571 -0.9 -0.88571429 -0.87142857 -0.85714286 -0.84285714 -0.82857143 -0.81428571 -0.8 -0.78571429 -0.77142857 -0.75714286 -0.74285714 -0.72857143 -0.71428571 -0.7 -0.68571429 -0.67142857 -0.65714286 -0.64285714 -0.62857143 -0.61428571 -0.6 -0.58571429 -0.57142857 -0.55714286 -0.54285714 -0.52857143 -0.51428571 -0.5 -0.48571429 -0.47142857 -0.45714286 -0.44285714 -0.42857143 -0.41428571 -0.4 -0.38571429 -0.37142857 -0.35714286 -0.34285714 -0.32857143 -0.31428571 -0.3 -0.28571429 -0.27142857 -0.25714286 -0.24285714 -0.22857143 -0.21428571 -0.2 -0.18571429 -0.17142857 -0.15714286 -0.14285714 -0.12857143 -0.11428571 -0.1 -0.08571429 -0.07142857 -0.06937658 -0.06937658 -0.06937658 -0.06937658 -0.06937658 -0.06937658
  spline S23 degree 3 poles (-20.7182, -1.1345) (-20.7189, -1.1215) (-20.7221, -1.1087) (-20.7333, -1.0852) (-20.7411, -1.0747) (-20.759, -1.0584) (-20.7684, -1.0524) (-20.7889, -1.0436) (-20.7998, -1.041) (-20.8108, -1.0402) knots 0 0 0 0 0.003906 0.003906 0.007813 0.007813 0.011148 0.011148 0.014483 0.014483 0.014483 0.014483
  arc A42 (-20.7182, -1.1345) -> (-20.6687, -1.8256) centre (0, 0) ccw
  spline S24 degree 3 poles (-20.7471, -1.9321) (-20.7343, -1.9293) (-20.7223, -1.9241) (-20.7008, -1.9093) (-20.6917, -1.8999) (-20.6785, -1.8796) (-20.674, -1.8694) (-20.6686, -1.8478) (-20.6678, -1.8366) (-20.6687, -1.8256) knots 0 0 0 0 0.003906 0.003906 0.007813 0.007813 0.011148 0.011148 0.014483 0.014483 0.014483 0.014483
  spline S25 degree 5 poles (-20.7471, -1.9321) (-20.748, -1.9323) (-20.7556, -1.9339) (-20.7698, -1.9371) (-20.7906, -1.9419) (-20.8179, -1.9485) (-20.8509, -1.9569) (-20.8838, -1.9657) (-20.9167, -1.9748) (-20.9495, -1.9842) (-20.9823, -1.9939) (-21.0151, -2.0039) (-21.0478, -2.0141) (-21.0804, -2.0245) (-21.113, -2.0352) (-21.1456, -2.0462) (-21.1782, -2.0575) (-21.2107, -2.069) (-21.2431, -2.0807) (-21.2755, -2.0926) (-21.3079, -2.1047) (-21.3403, -2.1171) (-21.3726, -2.1296) (-21.4048, -2.1424) (-21.4371, -2.1554) (-21.4693, -2.1686) (-21.5014, -2.1819) (-21.5335, -2.1955) (-21.5656, -2.2093) (-21.5976, -2.2232) (-21.6296, -2.2373) (-21.6616, -2.2517) (-21.6935, -2.2661) (-21.7254, -2.2808) (-21.7573, -2.2957) (-21.7891, -2.3107) (-21.8209, -2.3259) (-21.8526, -2.3412) (-21.8843, -2.3567) (-21.9159, -2.3724) (-21.9476, -2.3883) (-21.9792, -2.4043) (-22.0107, -2.4205) (-22.0422, -2.4368) (-22.0737, -2.4533) (-22.1051, -2.4699) (-22.1365, -2.4867) (-22.1679, -2.5037) (-22.1992, -2.5208) (-22.2305, -2.538) (-22.2617, -2.5554) (-22.2929, -2.573) (-22.3241, -2.5907) (-22.3552, -2.6085) (-22.3863, -2.6265) (-22.4173, -2.6447) (-22.4483, -2.6629) (-22.4793, -2.6814) (-22.5102, -2.6999) (-22.5411, -2.7186) (-22.572, -2.7374) (-22.6028, -2.7564) (-22.6336, -2.7755) (-22.6643, -2.7948) (-22.695, -2.8142) (-22.7256, -2.8337) (-22.7562, -2.8533) (-22.7807, -2.8692) (-22.799, -2.8811) (-22.8112, -2.8891) (-22.8173, -2.8931) knots 0.06937658 0.06937658 0.06937658 0.06937658 0.06937658 0.06937658 0.07142857 0.08571429 0.1 0.11428571 0.12857143 0.14285714 0.15714286 0.17142857 0.18571429 0.2 0.21428571 0.22857143 0.24285714 0.25714286 0.27142857 0.28571429 0.3 0.31428571 0.32857143 0.34285714 0.35714286 0.37142857 0.38571429 0.4 0.41428571 0.42857143 0.44285714 0.45714286 0.47142857 0.48571429 0.5 0.51428571 0.52857143 0.54285714 0.55714286 0.57142857 0.58571429 0.6 0.61428571 0.62857143 0.64285714 0.65714286 0.67142857 0.68571429 0.7 0.71428571 0.72857143 0.74285714 0.75714286 0.77142857 0.78571429 0.8 0.81428571 0.82857143 0.84285714 0.85714286 0.87142857 0.88571429 0.9 0.91428571 0.92857143 0.94285714 0.95714286 0.97142857 0.98571429 1 1 1 1 1 1
  arc A43 (-22.8173, -2.8931) -> (-22.7081, -3.6525) centre (0, 0) ccw
  spline S26 degree 5 poles (-22.7081, -3.6525) (-22.7011, -3.6546) (-22.6872, -3.6588) (-22.6662, -3.6651) (-22.6383, -3.6734) (-22.6034, -3.6837) (-22.5685, -3.6937) (-22.5336, -3.7037) (-22.4987, -3.7135) (-22.4638, -3.7232) (-22.4289, -3.7327) (-22.394, -3.7421) (-22.3591, -3.7513) (-22.3242, -3.7604) (-22.2893, -3.7694) (-22.2544, -3.7782) (-22.2195, -3.7868) (-22.1846, -3.7953) (-22.1497, -3.8037) (-22.1148, -3.8119) (-22.0799, -3.8199) (-22.045, -3.8278) (-22.0101, -3.8356) (-21.9753, -3.8432) (-21.9404, -3.8506) (-21.9056, -3.8579) (-21.8707, -3.865) (-21.8359, -3.8719) (-21.801, -3.8787) (-21.7662, -3.8854) (-21.7314, -3.8918) (-21.6966, -3.8981) (-21.6618, -3.9042) (-21.627, -3.9102) (-21.5922, -3.916) (-21.5575, -3.9216) (-21.5227, -3.9271) (-21.488, -3.9323) (-21.4532, -3.9374) (-21.4185, -3.9423) (-21.3838, -3.9471) (-21.3491, -3.9516) (-21.3145, -3.956) (-21.2798, -3.9601) (-21.2452, -3.9641) (-21.2106, -3.9679) (-21.176, -3.9714) (-21.1414, -3.9748) (-21.1068, -3.978) (-21.0723, -3.9809) (-21.0378, -3.9837) (-21.0033, -3.9862) (-20.9688, -3.9885) (-20.9344, -3.9906) (-20.9, -3.9924) (-20.8656, -3.9941) (-20.8312, -3.9954) (-20.7969, -3.9965) (-20.7626, -3.9974) (-20.7284, -3.9979) (-20.6941, -3.9983) (-20.6599, -3.9983) (-20.6258, -3.9981) (-20.5917, -3.9975) (-20.5576, -3.9967) (-20.5236, -3.9955) (-20.4955, -3.9941) (-20.4742, -3.9929) (-20.4597, -3.9919) (-20.452, -3.9914) (-20.451, -3.9913) knots -1 -1 -1 -1 -1 -1 -0.98571429 -0.97142857 -0.95714286 -0.94285714 -0.92857143 -0.91428571 -0.9 -0.88571429 -0.87142857 -0.85714286 -0.84285714 -0.82857143 -0.81428571 -0.8 -0.78571429 -0.77142857 -0.75714286 -0.74285714 -0.72857143 -0.71428571 -0.7 -0.68571429 -0.67142857 -0.65714286 -0.64285714 -0.62857143 -0.61428571 -0.6 -0.58571429 -0.57142857 -0.55714286 -0.54285714 -0.52857143 -0.51428571 -0.5 -0.48571429 -0.47142857 -0.45714286 -0.44285714 -0.42857143 -0.41428571 -0.4 -0.38571429 -0.37142857 -0.35714286 -0.34285714 -0.32857143 -0.31428571 -0.3 -0.28571429 -0.27142857 -0.25714286 -0.24285714 -0.22857143 -0.21428571 -0.2 -0.18571429 -0.17142857 -0.15714286 -0.14285714 -0.12857143 -0.11428571 -0.1 -0.08571429 -0.07142857 -0.06937658 -0.06937658 -0.06937658 -0.06937658 -0.06937658 -0.06937658
  spline S27 degree 3 poles (-20.3458, -4.0714) (-20.3484, -4.0587) (-20.3534, -4.0465) (-20.3678, -4.0248) (-20.3771, -4.0155) (-20.3971, -4.002) (-20.4073, -3.9973) (-20.4287, -3.9916) (-20.4399, -3.9905) (-20.451, -3.9913) knots 0 0 0 0 0.003906 0.003906 0.007813 0.007813 0.011148 0.011148 0.014483 0.014483 0.014483 0.014483
  arc A44 (-20.3458, -4.0714) -> (-20.1986, -4.7484) centre (0, 0) ccw
  spline S28 degree 3 poles (-20.2609, -4.865) (-20.2487, -4.8605) (-20.2375, -4.8536) (-20.2184, -4.8359) (-20.2107, -4.8252) (-20.2005, -4.8034) (-20.1975, -4.7926) (-20.1953, -4.7704) (-20.196, -4.7593) (-20.1986, -4.7484) knots 0 0 0 0 0.003906 0.003906 0.007813 0.007813 0.011148 0.011148 0.014483 0.014483 0.014483 0.014483
  spline S29 degree 5 poles (-20.2609, -4.865) (-20.2618, -4.8654) (-20.2691, -4.8681) (-20.2827, -4.8732) (-20.3026, -4.8809) (-20.3287, -4.8914) (-20.3602, -4.9044) (-20.3915, -4.9178) (-20.4227, -4.9315) (-20.4539, -4.9455) (-20.485, -4.9597) (-20.516, -4.9742) (-20.5469, -4.989) (-20.5777, -5.004) (-20.6085, -5.0192) (-20.6392, -5.0347) (-20.6698, -5.0505) (-20.7003, -5.0665) (-20.7308, -5.0827) (-20.7612, -5.0991) (-20.7915, -5.1157) (-20.8218, -5.1326) (-20.852, -5.1496) (-20.8821, -5.1668) (-20.9121, -5.1843) (-20.9421, -5.2019) (-20.972, -5.2197) (-21.0019, -5.2377) (-21.0317, -5.2559) (-21.0614, -5.2743) (-21.0911, -5.2928) (-21.1207, -5.3115) (-21.1502, -5.3304) (-21.1797, -5.3494) (-21.2091, -5.3687) (-21.2385, -5.3881) (-21.2677, -5.4076) (-21.297, -5.4273) (-21.3261, -5.4472) (-21.3552, -5.4672) (-21.3843, -5.4874) (-21.4133, -5.5078) (-21.4422, -5.5283) (-21.4711, -5.5489) (-21.4999, -5.5697) (-21.5286, -5.5907) (-21.5573, -5.6118) (-21.5859, -5.633) (-21.6145, -5.6544) (-21.643, -5.6759) (-21.6714, -5.6976) (-21.6998, -5.7194) (-21.7281, -5.7414) (-21.7564, -5.7635) (-21.7846, -5.7857) (-21.8128, -5.8081) (-21.8409, -5.8306) (-21.8689, -5.8532) (-21.8969, -5.876) (-21.9248, -5.8989) (-21.9526, -5.9219) (-21.9804, -5.9451) (-22.0082, -5.9684) (-22.0359, -5.9918) (-22.0635, -6.0153) (-22.091, -6.039) (-22.1185, -6.0628) (-22.1405, -6.082) (-22.1569, -6.0964) (-22.1679, -6.106) (-22.1733, -6.1109) knots 0.06937658 0.06937658 0.06937658 0.06937658 0.06937658 0.06937658 0.07142857 0.08571429 0.1 0.11428571 0.12857143 0.14285714 0.15714286 0.17142857 0.18571429 0.2 0.21428571 0.22857143 0.24285714 0.25714286 0.27142857 0.28571429 0.3 0.31428571 0.32857143 0.34285714 0.35714286 0.37142857 0.38571429 0.4 0.41428571 0.42857143 0.44285714 0.45714286 0.47142857 0.48571429 0.5 0.51428571 0.52857143 0.54285714 0.55714286 0.57142857 0.58571429 0.6 0.61428571 0.62857143 0.64285714 0.65714286 0.67142857 0.68571429 0.7 0.71428571 0.72857143 0.74285714 0.75714286 0.77142857 0.78571429 0.8 0.81428571 0.82857143 0.84285714 0.85714286 0.87142857 0.88571429 0.9 0.91428571 0.92857143 0.94285714 0.95714286 0.97142857 0.98571429 1 1 1 1 1 1
  arc A45 (-22.1733, -6.1109) -> (-21.9572, -6.847) centre (0, 0) ccw
  spline S30 degree 5 poles (-21.9572, -6.847) (-21.95, -6.8481) (-21.9356, -6.8503) (-21.9139, -6.8536) (-21.8851, -6.8578) (-21.8491, -6.863) (-21.8131, -6.868) (-21.7771, -6.8729) (-21.7412, -6.8776) (-21.7053, -6.8822) (-21.6694, -6.8867) (-21.6335, -6.891) (-21.5976, -6.8952) (-21.5618, -6.8992) (-21.5259, -6.9031) (-21.4901, -6.9068) (-21.4544, -6.9104) (-21.4186, -6.9139) (-21.3829, -6.9172) (-21.3472, -6.9203) (-21.3115, -6.9233) (-21.2759, -6.9262) (-21.2403, -6.9289) (-21.2047, -6.9314) (-21.1691, -6.9338) (-21.1336, -6.9361) (-21.0981, -6.9382) (-21.0626, -6.9401) (-21.0271, -6.9419) (-20.9917, -6.9435) (-20.9563, -6.9449) (-20.921, -6.9462) (-20.8857, -6.9473) (-20.8504, -6.9483) (-20.8151, -6.949) (-20.7799, -6.9497) (-20.7448, -6.9501) (-20.7096, -6.9504) (-20.6745, -6.9505) (-20.6395, -6.9504) (-20.6044, -6.9501) (-20.5695, -6.9497) (-20.5345, -6.9491) (-20.4996, -6.9482) (-20.4648, -6.9472) (-20.43, -6.9461) (-20.3952, -6.9447) (-20.3605, -6.9431) (-20.3259, -6.9413) (-20.2913, -6.9393) (-20.2567, -6.9371) (-20.2222, -6.9347) (-20.1878, -6.9321) (-20.1534, -6.9292) (-20.119, -6.9262) (-20.0848, -6.9229) (-20.0506, -6.9194) (-20.0164, -6.9156) (-19.9824, -6.9115) (-19.9484, -6.9072) (-19.9145, -6.9026) (-19.8806, -6.8978) (-19.8469, -6.8927) (-19.8132, -6.8874) (-19.7796, -6.8817) (-19.7461, -6.8756) (-19.7185, -6.8703) (-19.6975, -6.866) (-19.6833, -6.863) (-19.6757, -6.8614) (-19.6748, -6.8612) knots -1 -1 -1 -1 -1 -1 -0.98571429 -0.97142857 -0.95714286 -0.94285714 -0.92857143 -0.91428571 -0.9 -0.88571429 -0.87142857 -0.85714286 -0.84285714 -0.82857143 -0.81428571 -0.8 -0.78571429 -0.77142857 -0.75714286 -0.74285714 -0.72857143 -0.71428571 -0.7 -0.68571429 -0.67142857 -0.65714286 -0.64285714 -0.62857143 -0.61428571 -0.6 -0.58571429 -0.57142857 -0.55714286 -0.54285714 -0.52857143 -0.51428571 -0.5 -0.48571429 -0.47142857 -0.45714286 -0.44285714 -0.42857143 -0.41428571 -0.4 -0.38571429 -0.37142857 -0.35714286 -0.34285714 -0.32857143 -0.31428571 -0.3 -0.28571429 -0.27142857 -0.25714286 -0.24285714 -0.22857143 -0.21428571 -0.2 -0.18571429 -0.17142857 -0.15714286 -0.14285714 -0.12857143 -0.11428571 -0.1 -0.08571429 -0.07142857 -0.06937658 -0.06937658 -0.06937658 -0.06937658 -0.06937658 -0.06937658
  spline S31 degree 3 poles (-19.5593, -6.9255) (-19.5637, -6.9132) (-19.5704, -6.9019) (-19.5877, -6.8825) (-19.5982, -6.8746) (-19.6199, -6.8641) (-19.6307, -6.8609) (-19.6527, -6.8583) (-19.6639, -6.8588) (-19.6748, -6.8612) knots 0 0 0 0 0.003906 0.003906 0.007813 0.007813 0.011148 0.011148 0.014483 0.014483 0.014483 0.014483
  arc A46 (-19.5593, -6.9255) -> (-19.3172, -7.5747) centre (0, 0) ccw
  spline S32 degree 3 poles (-19.3623, -7.6989) (-19.3509, -7.6927) (-19.3408, -7.6843) (-19.3244, -7.664) (-19.3183, -7.6524) (-19.3113, -7.6293) (-19.3099, -7.6182) (-19.3108, -7.596) (-19.3131, -7.585) (-19.3172, -7.5747) knots 0 0 0 0 0.003906 0.003906 0.007813 0.007813 0.011148 0.011148 0.014483 0.014483 0.014483 0.014483
  spline S33 degree 5 poles (-19.3623, -7.6989) (-19.3632, -7.6994) (-19.37, -7.7031) (-19.3827, -7.7101) (-19.4013, -7.7206) (-19.4257, -7.7347) (-19.455, -7.7521) (-19.4841, -7.7698) (-19.513, -7.7878) (-19.5419, -7.806) (-19.5706, -7.8245) (-19.5993, -7.8433) (-19.6278, -7.8623) (-19.6561, -7.8816) (-19.6844, -7.901) (-19.7126, -7.9208) (-19.7406, -7.9407) (-19.7686, -7.9609) (-19.7964, -7.9813) (-19.8242, -8.0018) (-19.8518, -8.0226) (-19.8794, -8.0436) (-19.9068, -8.0647) (-19.9342, -8.0861) (-19.9615, -8.1076) (-19.9886, -8.1293) (-20.0157, -8.1512) (-20.0427, -8.1733) (-20.0696, -8.1955) (-20.0964, -8.2179) (-20.1232, -8.2405) (-20.1498, -8.2632) (-20.1763, -8.2861) (-20.2028, -8.3092) (-20.2292, -8.3324) (-20.2555, -8.3558) (-20.2817, -8.3793) (-20.3078, -8.403) (-20.3339, -8.4268) (-20.3598, -8.4508) (-20.3857, -8.4749) (-20.4115, -8.4991) (-20.4372, -8.5235) (-20.4628, -8.5481) (-20.4884, -8.5728) (-20.5138, -8.5976) (-20.5392, -8.6226) (-20.5645, -8.6477) (-20.5898, -8.6729) (-20.6149, -8.6983) (-20.64, -8.7238) (-20.665, -8.7494) (-20.6899, -8.7752) (-20.7147, -8.8011) (-20.7395, -8.8271) (-20.7642, -8.8532) (-20.7888, -8.8795) (-20.8133, -8.9059) (-20.8378, -8.9324) (-20.8621, -8.9591) (-20.8864, -8.9858) (-20.9106, -9.0127) (-20.9348, -9.0397) (-20.9588, -9.0668) (-20.9828, -9.0941) (-21.0067, -9.1214) (-21.0306, -9.1489) (-21.0496, -9.171) (-21.0638, -9.1876) (-21.0733, -9.1987) (-21.078, -9.2043) knots 0.06937658 0.06937658 0.06937658 0.06937658 0.06937658 0.06937658 0.07142857 0.08571429 0.1 0.11428571 0.12857143 0.14285714 0.15714286 0.17142857 0.18571429 0.2 0.21428571 0.22857143 0.24285714 0.25714286 0.27142857 0.28571429 0.3 0.31428571 0.32857143 0.34285714 0.35714286 0.37142857 0.38571429 0.4 0.41428571 0.42857143 0.44285714 0.45714286 0.47142857 0.48571429 0.5 0.51428571 0.52857143 0.54285714 0.55714286 0.57142857 0.58571429 0.6 0.61428571 0.62857143 0.64285714 0.65714286 0.67142857 0.68571429 0.7 0.71428571 0.72857143 0.74285714 0.75714286 0.77142857 0.78571429 0.8 0.81428571 0.82857143 0.84285714 0.85714286 0.87142857 0.88571429 0.9 0.91428571 0.92857143 0.94285714 0.95714286 0.97142857 0.98571429 1 1 1 1 1 1
  arc A47 (-21.078, -9.2043) -> (-20.7593, -9.9022) centre (0, 0) ccw
  spline S34 degree 5 poles (-20.7593, -9.9022) (-20.752, -9.9022) (-20.7374, -9.9024) (-20.7155, -9.9025) (-20.6864, -9.9026) (-20.65, -9.9026) (-20.6137, -9.9024) (-20.5774, -9.9021) (-20.5411, -9.9017) (-20.5049, -9.9011) (-20.4687, -9.9004) (-20.4326, -9.8996) (-20.3965, -9.8986) (-20.3604, -9.8975) (-20.3244, -9.8963) (-20.2885, -9.8949) (-20.2525, -9.8934) (-20.2167, -9.8917) (-20.1808, -9.8899) (-20.145, -9.8879) (-20.1093, -9.8858) (-20.0736, -9.8836) (-20.038, -9.8812) (-20.0024, -9.8786) (-19.9668, -9.8759) (-19.9313, -9.8731) (-19.8959, -9.8701) (-19.8605, -9.867) (-19.8252, -9.8637) (-19.7899, -9.8602) (-19.7547, -9.8566) (-19.7195, -9.8529) (-19.6844, -9.8489) (-19.6493, -9.8449) (-19.6143, -9.8406) (-19.5794, -9.8362) (-19.5445, -9.8316) (-19.5097, -9.8269) (-19.4749, -9.822) (-19.4402, -9.8169) (-19.4056, -9.8117) (-19.3711, -9.8063) (-19.3366, -9.8007) (-19.3021, -9.7949) (-19.2678, -9.789) (-19.2335, -9.7828) (-19.1993, -9.7765) (-19.1652, -9.77) (-19.1311, -9.7633) (-19.0972, -9.7564) (-19.0633, -9.7493) (-19.0295, -9.742) (-18.9957, -9.7345) (-18.9621, -9.7268) (-18.9286, -9.7189) (-18.8951, -9.7108) (-18.8618, -9.7024) (-18.8285, -9.6938) (-18.7954, -9.685) (-18.7624, -9.6759) (-18.7294, -9.6665) (-18.6966, -9.6569) (-18.6639, -9.6471) (-18.6313, -9.637) (-18.5989, -9.6266) (-18.5666, -9.6158) (-18.54, -9.6066) (-18.5199, -9.5994) (-18.5063, -9.5944) (-18.499, -9.5917) (-18.4981, -9.5913) knots -1 -1 -1 -1 -1 -1 -0.98571429 -0.97142857 -0.95714286 -0.94285714 -0.92857143 -0.91428571 -0.9 -0.88571429 -0.87142857 -0.85714286 -0.84285714 -0.82857143 -0.81428571 -0.8 -0.78571429 -0.77142857 -0.75714286 -0.74285714 -0.72857143 -0.71428571 -0.7 -0.68571429 -0.67142857 -0.65714286 -0.64285714 -0.62857143 -0.61428571 -0.6 -0.58571429 -0.57142857 -0.55714286 -0.54285714 -0.52857143 -0.51428571 -0.5 -0.48571429 -0.47142857 -0.45714286 -0.44285714 -0.42857143 -0.41428571 -0.4 -0.38571429 -0.37142857 -0.35714286 -0.34285714 -0.32857143 -0.31428571 -0.3 -0.28571429 -0.27142857 -0.25714286 -0.24285714 -0.22857143 -0.21428571 -0.2 -0.18571429 -0.17142857 -0.15714286 -0.14285714 -0.12857143 -0.11428571 -0.1 -0.08571429 -0.07142857 -0.06937658 -0.06937658 -0.06937658 -0.06937658 -0.06937658 -0.06937658
  spline S35 degree 3 poles (-18.3746, -9.6386) (-18.3807, -9.6271) (-18.3889, -9.6168) (-18.4089, -9.6001) (-18.4204, -9.5937) (-18.4434, -9.5864) (-18.4545, -9.5848) (-18.4767, -9.5853) (-18.4877, -9.5875) (-18.4981, -9.5913) knots 0 0 0 0 0.003906 0.003906 0.007813 0.007813 0.011148 0.011148 0.014483 0.014483 0.014483 0.014483
  arc A48 (-18.3746, -9.6386) -> (-18.0426, -10.2467) centre (0, 0) ccw
  spline S36 degree 3 poles (-18.0696, -10.3761) (-18.0592, -10.3683) (-18.0504, -10.3585) (-18.037, -10.3362) (-18.0326, -10.3238) (-18.029, -10.2999) (-18.0292, -10.2887) (-18.0332, -10.2669) (-18.0371, -10.2564) (-18.0426, -10.2467) knots 0 0 0 0 0.003906 0.003906 0.007813 0.007813 0.011148 0.011148 0.014483 0.014483 0.014483 0.014483
  spline S37 degree 5 poles (-18.0696, -10.3761) (-18.0704, -10.3767) (-18.0766, -10.3813) (-18.0882, -10.3901) (-18.1051, -10.4031) (-18.1272, -10.4205) (-18.1537, -10.4419) (-18.18, -10.4635) (-18.2061, -10.4855) (-18.2321, -10.5077) (-18.2579, -10.5301) (-18.2835, -10.5527) (-18.3091, -10.5756) (-18.3344, -10.5987) (-18.3596, -10.622) (-18.3847, -10.6455) (-18.4096, -10.6693) (-18.4344, -10.6932) (-18.4591, -10.7173) (-18.4836, -10.7417) (-18.508, -10.7662) (-18.5323, -10.7908) (-18.5565, -10.8157) (-18.5805, -10.8407) (-18.6045, -10.8659) (-18.6283, -10.8913) (-18.652, -10.9168) (-18.6755, -10.9425) (-18.699, -10.9683) (-18.7223, -10.9943) (-18.7456, -11.0204) (-18.7687, -11.0467) (-18.7917, -11.0732) (-18.8147, -11.0998) (-18.8375, -11.1265) (-18.8602, -11.1534) (-18.8828, -11.1804) (-18.9052, -11.2075) (-18.9276, -11.2348) (-18.9499, -11.2622) (-18.9721, -11.2898) (-18.9942, -11.3175) (-19.0161, -11.3453) (-19.038, -11.3732) (-19.0598, -11.4013) (-19.0815, -11.4295) (-19.1031, -11.4578) (-19.1245, -11.4863) (-19.1459, -11.5149) (-19.1672, -11.5435) (-19.1884, -11.5724) (-19.2095, -11.6013) (-19.2305, -11.6303) (-19.2514, -11.6595) (-19.2722, -11.6888) (-19.2929, -11.7182) (-19.3135, -11.7477) (-19.334, -11.7773) (-19.3544, -11.807) (-19.3748, -11.8369) (-19.395, -11.8668) (-19.4152, -11.8969) (-19.4352, -11.927) (-19.4552, -11.9573) (-19.475, -11.9877) (-19.4948, -12.0182) (-19.5145, -12.0488) (-19.5302, -12.0733) (-19.5419, -12.0918) (-19.5497, -12.1041) (-19.5535, -12.1103) knots 0.06937658 0.06937658 0.06937658 0.06937658 0.06937658 0.06937658 0.07142857 0.08571429 0.1 0.11428571 0.12857143 0.14285714 0.15714286 0.17142857 0.18571429 0.2 0.21428571 0.22857143 0.24285714 0.25714286 0.27142857 0.28571429 0.3 0.31428571 0.32857143 0.34285714 0.35714286 0.37142857 0.38571429 0.4 0.41428571 0.42857143 0.44285714 0.45714286 0.47142857 0.48571429 0.5 0.51428571 0.52857143 0.54285714 0.55714286 0.57142857 0.58571429 0.6 0.61428571 0.62857143 0.64285714 0.65714286 0.67142857 0.68571429 0.7 0.71428571 0.72857143 0.74285714 0.75714286 0.77142857 0.78571429 0.8 0.81428571 0.82857143 0.84285714 0.85714286 0.87142857 0.88571429 0.9 0.91428571 0.92857143 0.94285714 0.95714286 0.97142857 0.98571429 1 1 1 1 1 1
  arc A49 (-19.5535, -12.1103) -> (-19.1387, -12.7557) centre (0, 0) ccw
  spline S38 degree 5 poles (-19.1387, -12.7557) (-19.1315, -12.7548) (-19.1171, -12.7528) (-19.0954, -12.7498) (-19.0665, -12.7458) (-19.0305, -12.7406) (-18.9946, -12.7352) (-18.9587, -12.7298) (-18.9229, -12.7242) (-18.8871, -12.7185) (-18.8514, -12.7127) (-18.8158, -12.7067) (-18.7802, -12.7006) (-18.7446, -12.6944) (-18.7092, -12.688) (-18.6738, -12.6815) (-18.6384, -12.6749) (-18.6032, -12.6681) (-18.5679, -12.6612) (-18.5328, -12.6542) (-18.4977, -12.647) (-18.4627, -12.6397) (-18.4278, -12.6323) (-18.3929, -12.6247) (-18.3581, -12.617) (-18.3234, -12.6091) (-18.2887, -12.6011) (-18.2541, -12.593) (-18.2196, -12.5847) (-18.1852, -12.5763) (-18.1509, -12.5677) (-18.1166, -12.5589) (-18.0824, -12.5501) (-18.0483, -12.541) (-18.0142, -12.5319) (-17.9803, -12.5225) (-17.9464, -12.513) (-17.9126, -12.5034) (-17.8789, -12.4936) (-17.8453, -12.4836) (-17.8117, -12.4735) (-17.7783, -12.4633) (-17.745, -12.4528) (-17.7117, -12.4422) (-17.6786, -12.4314) (-17.6455, -12.4205) (-17.6125, -12.4094) (-17.5797, -12.3981) (-17.5469, -12.3866) (-17.5143, -12.3749) (-17.4818, -12.3631) (-17.4493, -12.351) (-17.417, -12.3388) (-17.3848, -12.3264) (-17.3527, -12.3138) (-17.3208, -12.301) (-17.289, -12.288) (-17.2573, -12.2747) (-17.2258, -12.2612) (-17.1944, -12.2475) (-17.1631, -12.2336) (-17.132, -12.2194) (-17.101, -12.205) (-17.0702, -12.1904) (-17.0396, -12.1755) (-17.0092, -12.1602) (-16.9841, -12.1473) (-16.9653, -12.1374) (-16.9525, -12.1304) (-16.9457, -12.1267) (-16.9448, -12.1263) knots -1 -1 -1 -1 -1 -1 -0.98571429 -0.97142857 -0.95714286 -0.94285714 -0.92857143 -0.91428571 -0.9 -0.88571429 -0.87142857 -0.85714286 -0.84285714 -0.82857143 -0.81428571 -0.8 -0.78571429 -0.77142857 -0.75714286 -0.74285714 -0.72857143 -0.71428571 -0.7 -0.68571429 -0.67142857 -0.65714286 -0.64285714 -0.62857143 -0.61428571 -0.6 -0.58571429 -0.57142857 -0.55714286 -0.54285714 -0.52857143 -0.51428571 -0.5 -0.48571429 -0.47142857 -0.45714286 -0.44285714 -0.42857143 -0.41428571 -0.4 -0.38571429 -0.37142857 -0.35714286 -0.34285714 -0.32857143 -0.31428571 -0.3 -0.28571429 -0.27142857 -0.25714286 -0.24285714 -0.22857143 -0.21428571 -0.2 -0.18571429 -0.17142857 -0.15714286 -0.14285714 -0.12857143 -0.11428571 -0.1 -0.08571429 -0.07142857 -0.06937658 -0.06937658 -0.06937658 -0.06937658 -0.06937658 -0.06937658
  spline S39 degree 3 poles (-16.8159, -12.1555) (-16.8235, -12.1449) (-16.8331, -12.136) (-16.8552, -12.1222) (-16.8675, -12.1176) (-16.8914, -12.1136) (-16.9025, -12.1136) (-16.9245, -12.1173) (-16.9351, -12.1209) (-16.9448, -12.1263) knots 0 0 0 0 0.003906 0.003906 0.007813 0.007813 0.011148 0.011148 0.014483 0.014483 0.014483 0.014483
  arc A50 (-16.8159, -12.1555) -> (-16.4007, -12.7101) centre (0, 0) ccw
  spline S40 degree 3 poles (-16.409, -12.8421) (-16.3998, -12.8329) (-16.3925, -12.8219) (-16.3824, -12.7979) (-16.3798, -12.785) (-16.3796, -12.7609) (-16.3814, -12.7498) (-16.3886, -12.7288) (-16.3939, -12.7189) (-16.4007, -12.7101) knots 0 0 0 0 0.003906 0.003906 0.007813 0.007813 0.011148 0.011148 0.014483 0.014483 0.014483 0.014483